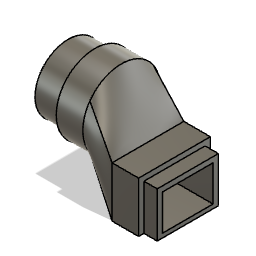
adapter v1 (Autodesk Fusion 360 design; units mm, degrees)
Autodesk Fusion 360 part; units mm, degrees
note: some values were not read from the file. Chosen so that the rebuilt part matches the saved one: which sketch regions a step uses.
ref_plane "WorkPlane1" through (-58, 27.9344, 0) normal (-1, 0, 0) x (0, 0, -1)
sketch "Sketch3" plane through (-58, 27.9344, 0) normal (-1, 0, 0) x (0, 0, -1)
  line L0 (11.5, 27.9344) -> (11.5, 10.9344)
  line L1 (-11.5, 10.9344) -> (11.5, 10.9344)
  line L2 (-11.5, 10.9344) -> (-11.5, 27.9344)
  line L3 (-11.5, 27.9344) -> (11.5, 27.9344)
  line L4 (13.5, 27.9344) -> (13.5, 8.9344)
  line L5 (-13.5, 8.9344) -> (13.5, 8.9344)
  line L6 (-13.5, 8.9344) -> (-13.5, 27.9344)
  line L7 (9.5, 27.9344) -> (9.5, 12.9344)
  line L8 (-9.5, 12.9344) -> (9.5, 12.9344)
  line L9 (-9.5, 12.9344) -> (-9.5, 27.9344)
  line L10 (13.5, 27.9344) -> (11.5, 27.9344)
  line L11 (-9.5, 27.9344) -> (-11.5, 27.9344)
  line L12 (-13.5, 27.9344) -> (-11.5, 27.9344)
  line L13 (9.5, 27.9344) -> (-9.5, 27.9344)
  line L14 (9.5, 26.3692) -> (-9.5, 26.3692)
  dimension "d92" = -2
  dimension "d93" = 2
  constraint coincident L0.start L3.end
  constraint perpendicular L0 L10
  constraint coincident L2.end L3.start
  constraint perpendicular L2 L11
  constraint perpendicular L2 L12
  constraint perpendicular L9 L13
  constraint coincident L7 L14.start
  constraint coincident L9 L14.end
  constraint perpendicular L9 L14
extrude "Extrude1" add sketch "Sketch3" against normal blind 5 contours L0 L1 L2 L3 L7 L8 L9 L11 | L3 L7 L9 L13 L14 makes body 1
extrude "Extrude2" add sketch "Sketch3" along normal blind 10 contours L0 L1 L2 L4 L5 L6 L10 L12 | L0 L1 L2 L3 L7 L8 L9 L11 | L3 L7 L9 L13 L14 bodies 1
ref_plane "WorkPlane2" through (-88, 27.9344, 0) normal (-1, 0, 0) x (0, 0, -1)
sketch "Sketch4" plane through (-88, 27.9344, 0) normal (-1, 0, 0) x (0, 0, -1)
  line L0 (-58, 27.9344) -> (58, 27.9344)
  circle A0 centre (0, 2.9344) radius 12.5
  circle A1 centre (0, 2.9344) radius 10.5
  circle A2 centre (0, 2.9344) radius 14.5
  dimension "d99" = 25
  dimension "d100" = 25
  dimension "d101" = 21
  dimension "d102" = 29
  constraint concentric A0 A1
  constraint concentric A0 A2
  measures "d99" diameter of A0
  measures "d100" distance of L0 A0.centre
  measures "d101" diameter of A1
  measures "d102" diameter of A2
extrude "Extrude3" add sketch "Sketch4" along normal blind 10 separate body contours A0 makes body 2
extrude "Extrude4" add sketch "Sketch4" against normal blind 10 contours A0 | A2 bodies 2
sketch "Sketch5" plane through (-68, 0, 0) normal (-1, 0, 0) x (0, 0, 1)
  line L0 (-9.5, 15) -> (9.5, 15)
  line L1 (9.5, 15) -> (9.5, 1.5652)
  line L2 (9.5, 1.5652) -> (-9.5, 1.5652)
  line L3 (-9.5, 1.5652) -> (-9.5, 15)
  line L4 (-13.5, 0) -> (13.5, 0)
  line L5 (13.5, 0) -> (13.5, 19)
  line L6 (13.5, 19) -> (-13.5, 19)
  line L7 (-13.5, 19) -> (-13.5, 0)
  line L8 (13.5, 19) -> (-13.5, 19)
  line L9 (-13.5, 0) -> (-13.5, 19)
  line L10 (13.5, 19) -> (13.5, 0)
  line L11 (11.5, 0) -> (-11.5, 0)
sketch "Sketch6" plane through (-78, 0, 0) normal (1, 0, 0) x (0, 0, -1)
  circle A0 centre (0, 25) radius 10.5
  circle A1 centre (0, 25) radius 14.5
  circle A2 centre (0, 25) radius 14.5
loft "Loft1" add profiles "Sketch6", "Sketch5" section 1 contours A0 | A1 A2 section 2 bodies 1 2
loft "Loft2" cut section 1 face at (-78, 28.7681, -1.1623) section 2 face at (-68, 6.0434, -3.1667) on bodies 1 bodies 1
named bodies: "ADAPTER"
